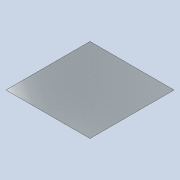
# Autodesk Inventor part: Podłoga
Saved by Autodesk Inventor 2021.3 (Build 253353000, 353)
## iProperties
Created: 2023-05-23
Part Number: Podłoga
Material: Ogólny
Document SubType Name: Modeling
Designer: User
Density: 1 g/cm^3
Appearance: Dżins — niebieski
Author: User
Autodesk Inventor part; units mm, degrees
ref_plane "YZ Plane" through (0, 0, 0) normal (1, 0, 0) x (0, 1, 0)
ref_plane "XZ Plane" through (0, 0, 0) normal (0, 1, 0) x (-1, 0, 0)
ref_plane "XY Plane" through (0, 0, 0) normal (0, 0, 1) x (1, 0, 0)
sketch "Szkic1" plane through (0, 0, 0) normal (0, 1, 0) x (-1, 0, 0)
  line L0 (57419.3548, 47419.3547) -> (47419.3548, 47419.3547)
  line L1 (47419.3548, 47419.3547) -> (47419.3548, 37419.3547)
  line L2 (47419.3548, 37419.3547) -> (57419.3548, 37419.3547)
  line L3 (57419.3548, 37419.3547) -> (57419.3548, 47419.3547)
  point P0 (0, 0)
  dimension "d0" = 10000
  dimension "d1" = 10000
  constraints: 8 end point, 2 parallel, 1 horizontal, 1 perpendicular
  measures "d0" distance of L1.end L2.end
  measures "d1" distance of L2.end L0.start
extrude "Wyciągnięcie proste1" add sketch "Szkic1" along normal blind 1
